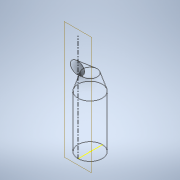
# Autodesk Inventor part: Pièce1
Saved by Autodesk Inventor 2020 (Build 240168000, 168)
## iProperties
Created: 2023-09-30
Part Number: Pièce1
Material: Générique
Document SubType Name: Modeling
Designer: Admin
Density: 1 g/cm^3
Appearance: Par défaut
Author: Admin
Autodesk Inventor part; units mm, degrees
ref_plane "YZ Plane" through (0, 0, 0) normal (1, 0, 0) x (0, 1, 0)
ref_plane "XZ Plane" through (0, 0, 0) normal (0, 1, 0) x (-1, 0, 0)
sketch "Esquisse1" plane through (0, 0, 0) normal (0, 1, 0) x (-1, 0, 0)
  circle A0 centre (0, 0) radius 11.857
  circle A1 centre (0, 0) radius 11.357
  dimension "d0" = 23.714
  dimension "d1" = 0.5
  constraints: 2 centre point, 2 coincident
  measures "d0" diameter of A0
  measures "d1" radial gap between concentric circles of A0 A1
extrude "Extrusion1" add sketch "Esquisse1" along normal blind 50
sketch "Esquisse3" plane through (0, 0, 0) normal (1, 0, 0) x (0, 1, 0)
  line L0 (50, -11.857) -> (50, 11.857) projected
  line L1 (50, -11.857) -> (50, -11.357)
  line L2 (50, -11.857) -> (65.1546, -6.9812)
  line L3 (65.1546, -6.9812) -> (65.1546, -6.5993)
  line L4 (65.1546, -6.5993) -> (50, -11.357)
  point P0 (0, 0)
  constraints: 8 end point, 1 parallel, 1 point on line
sketch "Esquisse4" plane through (0, 0, 0) normal (1, 0, 0) x (0, 1, 0)
  line L0 (89.7518, 0) -> (0, 0)
  line L1 (50, -11.857) -> (50, 11.857) projected
  line L2 (65.5189, 0) -> (87.7272, 26.0465)
  constraints: 4 end point, 1 horizontal, 1 point on line
revolve "Révolution1" add sketch "Esquisse3" angle 360 about axis through (0, 89.7518, 0) along (0, -1, 0)
sketch "Esquisse6" plane through (0, 0, 0) normal (1, 0, 0) x (0, 1, 0)
  line L0 (0, -11.857) -> (0, 11.857) projected
  line L1 (0, 11.857) -> (102.0428, 11.857)
  point P0 (0, 0)
  constraints: 2 end point, 1 horizontal
ref_plane "Plan de construction1" through (0, 0, 11.857) normal (0, 0, 1) x (1, 0, 0)
sketch "Esquisse10" plane through (0, 65.1546, 0) normal (0, 1, 0) x (1, 0, 0)
  circle A0 centre (0, 0) radius 6.5993
  circle A1 centre (0, 0) radius 6.9812
  constraints: 2 centre point, 2 coincident
sweep "Balayage1" add profiles "Esquisse10" path "Esquisse4" path curves L2
sketch "Esquisse13" plane through (0, 0, 0) normal (1, 0, 0) x (0, 1, 0)
  line L0 (101.04, 12.0731) -> (64.1022, 12.0731)
  line L1 (64.1022, 12.0731) -> (64.1022, 38.95)
  line L2 (64.1022, 38.95) -> (101.04, 38.95)
  line L3 (101.04, 38.95) -> (101.04, 12.0731)
  point P0 (0, 0)
  constraints: 8 end point, 2 parallel, 1 horizontal, 1 perpendicular
extrude "Extrusion2" cut sketch "Esquisse13" against normal mid plane 50
